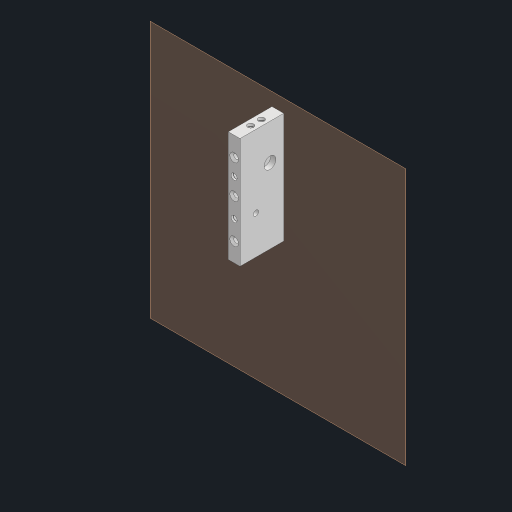
# Autodesk Inventor part: middle_gear_holder
Saved by Autodesk Inventor 2023 (Build 270158000, 158)
## iProperties
Created: 2024-04-23
Part Number: middle_gear_holder
Material: Generic
Document SubType Name: Modeling
Designer: szymo
Density: 1 g/cm^3
Appearance: Default
Author: szymo
Autodesk Inventor part; units mm, degrees
ref_plane "YZ Plane" through (0, 0, 0) normal (1, 0, 0) x (0, 1, 0)
ref_plane "XZ Plane" through (0, 0, 0) normal (0, 1, 0) x (-1, 0, 0)
ref_plane "Work Plane1" through (0, 0, 0) normal (0, 0, 1) x (1, 0, 0)
ref_plane "Work Plane2" through (-89, -40.3889, 33.5) normal (0, 0, 1) x (1, 0, 0)
sketch "Sketch1" plane through (0, 0, 0) normal (0, 0, 1) x (1, 0, 0)
  line L0 (23.5, 88.5) -> (-23.5, 88.5) projected
  line L1 (-23.5, 88.5) -> (-23.5, 36.5) projected
  line L2 (-26.5, 33.5) -> (-89, 33.5) projected
  line L3 (-89, 33.5) -> (-89, -72.5) projected
  line L4 (-89, -72.5) -> (-77, -72.5) projected
  line L5 (-74, -75.5) -> (-74, -93.5) projected
  line L6 (-74, -93.5) -> (74, -93.5) projected
  line L7 (74, -93.5) -> (74, -75.5) projected
  line L8 (77, -72.5) -> (89, -72.5) projected
  line L9 (89, -72.5) -> (89, 33.5) projected
  line L10 (89, 33.5) -> (26.5, 33.5) projected
  line L11 (23.5, 36.5) -> (23.5, 88.5) projected
  line L12 (-4.5, 81.5) -> (-4.5, 36.5) projected
  line L13 (-7.5, 33.5) -> (-13.5, 33.5) projected
  line L14 (-16.5, 36.5) -> (-16.5, 81.5) projected
  line L15 (-13.5, 84.5) -> (-7.5, 84.5) projected
  line L16 (16.5, 81.5) -> (16.5, 36.5) projected
  line L17 (13.5, 33.5) -> (7.5, 33.5) projected
  line L18 (4.5, 36.5) -> (4.5, 81.5) projected
  line L19 (7.5, 84.5) -> (13.5, 84.5) projected
  line L20 (-4.5, 88.5) -> (4.5, 88.5)
  line L21 (4.5, 88.5) -> (4.5, 3.75)
  line L22 (4.5, 3.75) -> (-4.5, 3.75)
  line L23 (-4.5, 3.75) -> (-4.5, 88.5)
  line L24 (-32.2, 4.75) -> (-59.9, 4.75)
  arc A0 (13.5, 33.5) -> (16.5, 36.5) centre (13.5, 36.5) ccw projected
  arc A1 (4.5, 36.5) -> (7.5, 33.5) centre (7.5, 36.5) ccw projected
  arc A2 (7.5, 84.5) -> (4.5, 81.5) centre (7.5, 81.5) ccw projected
  arc A3 (16.5, 81.5) -> (13.5, 84.5) centre (13.5, 81.5) ccw projected
  arc A4 (-4.5, 81.5) -> (-7.5, 84.5) centre (-7.5, 81.5) ccw projected
  arc A5 (-7.5, 33.5) -> (-4.5, 36.5) centre (-7.5, 36.5) ccw projected
  arc A6 (-16.5, 36.5) -> (-13.5, 33.5) centre (-13.5, 36.5) ccw projected
  arc A7 (-13.5, 84.5) -> (-16.5, 81.5) centre (-13.5, 81.5) ccw projected
  arc A8 (-26.5, 33.5) -> (-23.5, 36.5) centre (-26.5, 36.5) ccw projected
  arc A9 (-74, -75.5) -> (-77, -72.5) centre (-77, -75.5) ccw projected
  arc A10 (77, -72.5) -> (74, -75.5) centre (77, -75.5) ccw projected
  arc A11 (23.5, 36.5) -> (26.5, 33.5) centre (26.5, 36.5) ccw projected
  point P0 (0, 0)
  point P1 (-4.5, 81.5)
  point P2 (-4.5, 36.5)
  dimension "d0" = 1
  constraints: 10 end point, 2 collinear, 2 horizontal, 2 parallel, 1 perpendicular, 1 point on line, 2 other
  measures "d0" distance between parallel lines of L24 L22
extrude "Extrusion1" add sketch "Sketch1" along normal up to surface (33.5 mm away) contours L21 L18 L22 L23 L12 L0
sketch "Sketch2" plane through (4.5, 3.75, 0) normal (1, 0, 0) x (0, 0, -1)
  circle A0 centre (-21.2694, 29.2497) radius 2 projected
  point P0 (0, -3.75)
extrude "Extrusion2" cut sketch "Sketch2" against normal blind 10
sketch "Sketch3" plane through (4.5, 3.75, 0) normal (1, 0, 0) x (0, 0, -1)
  circle A0 centre (-10.5, 57.25) radius 4.5 projected
  point P0 (0, -3.75)
extrude "Extrusion3" cut sketch "Sketch3" against normal blind 4
sketch "Sketch4" plane through (-4.5, 3.75, 0) normal (-1, 0, 0) x (0, 0, 1)
  circle A0 centre (10.5, 57.25) radius 4.5 projected
  point P0 (0, -3.75)
extrude "Extrusion4" cut sketch "Sketch4" against normal blind 4
sketch "Sketch5" plane through (-4.5, 3.75, 33.5) normal (0, 0, 1) x (1, 0, 0)
  line L0 (5, 61.75) -> (5, 52.75) projected
  line L1 (4, 52.75) -> (4, 61.75) projected
  line L2 (9, 27.2497) -> (0, 27.2497) projected
  line L3 (9, 31.2497) -> (0, 31.2497) projected
  line L4 (17, 78.15) -> (-8, 78.15)
  line L5 (-8, 35.85) -> (17, 35.85)
  line L6 (9, 84.75) -> (9, 0) projected
  line L7 (0, 52.75) -> (0, 61.75) projected
  line L8 (9, 35.85) -> (0, 35.85)
  line L9 (0, 35.85) -> (0, 52.75)
  line L10 (0, 52.75) -> (9, 52.75)
  line L11 (9, 52.75) -> (9, 35.85)
  line L12 (0, 0) -> (0, 84.75) projected
  line L13 (9, 78.15) -> (0, 78.15)
  line L14 (0, 78.15) -> (0, 61.75)
  line L15 (0, 61.75) -> (9, 61.75)
  line L16 (9, 61.75) -> (9, 78.15)
  line L17 (-18, 7.625) -> (-18, 21.125) projected
  line L18 (-18, 14.375) -> (27, 14.375)
  line L19 (9, 35.85) -> (0, 52.75)
  line L20 (9, 61.75) -> (9, 52.75) projected
  line L21 (0, 35.85) -> (9, 52.75)
  line L22 (9, 61.75) -> (0, 78.15)
  line L23 (0, 61.75) -> (9, 78.15)
  point P0 (4.5, -3.75)
  point P1 (4.5, 14.375)
  point P2 (4.5, 44.3)
  point P3 (4.5, 69.95)
  dimension "d9" = 4.5
  dimension "d10" = 4.5
  constraints: 30 end point, 5 horizontal, 5 point on line, 4 midpoint, 4 parallel, 2 perpendicular, 4 other
  measures "d9" distance from line of L6 point (4.5, 14.375)
  measures "d10" distance from line of point (4.5, 14.375) L12
hole "Hole1" at (0, 18.125, 33.5) at (0, 48.05, 33.5) at (0, 73.7, 33.5) direction (0, 0, -1) diameter 3.6 end through all countersink diameter 6.6 countersink angle 90 clearance for "Countersunk Flat Head Screw ISO 2009/7046" size "M3" standard "ISO"
sketch "Sketch6" plane through (-4.5, 3.75, 0) normal (0, -1, 0) x (1, 0, 0)
  line L0 (9, 33.5) -> (0, 33.5) projected
  line L1 (0, 0) -> (0, 33.5) projected
  line L2 (0, 0) -> (9, 0) projected
  line L3 (9, 0) -> (9, 33.5) projected
  line L4 (0, 16.75) -> (9, 16.75)
  line L5 (9, 16.75) -> (0, 33.5)
  line L6 (9, 33.5) -> (0, 16.75)
  line L7 (0, 16.75) -> (9, 0)
  line L8 (9, 16.75) -> (0, 0)
  point P0 (4.5, 0)
  point P1 (4.5, 8.375)
  point P2 (4.5, 25.125)
  constraints: 10 end point, 4 midpoint, 2 parallel
hole "Hole2" at (0, 3.75, 8.375) at (0, 3.75, 25.125) direction (0, 1, 0) diameter 4 depth 5.35 counterbore diameter 4.6 counterbore depth 0.75
sketch "Sketch7" plane through (-4.5, 88.5, 0) normal (0, 1, 0) x (1, 0, 0)
  line L0 (0, -33.5) -> (9, -33.5) projected
  line L1 (0, -33.5) -> (9, -33.5) projected
  line L2 (9, 0) -> (9, -33.5) projected
  line L3 (9, 0) -> (0, 0) projected
  line L4 (0, 0) -> (0, -33.5) projected
  line L5 (-8, -1.4) -> (-8, -6.6) projected
  line L6 (-8, -32.1) -> (-8, -26.9) projected
  line L7 (17, -32.1) -> (17, -26.9) projected
  line L8 (17, -1.4) -> (17, -6.6) projected
  line L9 (17, -32.1) -> (-8, -32.1)
  line L10 (-8, -32.1) -> (-8, -26.9)
  line L11 (-8, -26.9) -> (17, -26.9)
  line L12 (17, -26.9) -> (17, -32.1)
  line L13 (-8, -6.6) -> (17, -6.6)
  line L14 (17, -6.6) -> (17, -1.4)
  line L15 (17, -1.4) -> (-8, -1.4)
  line L16 (-8, -1.4) -> (-8, -6.6)
  line L17 (17, -6.6) -> (-8, -6.6)
  line L18 (-8, -6.6) -> (-8, -8.6)
  line L19 (-8, -8.6) -> (17, -8.6)
  line L20 (17, -8.6) -> (17, -6.6)
  line L21 (-8, -26.9) -> (17, -26.9)
  line L22 (17, -26.9) -> (17, -24.9)
  line L23 (17, -24.9) -> (-8, -24.9)
  line L24 (-8, -24.9) -> (-8, -26.9)
  line L25 (9, 0) -> (9, -33.5) projected
  line L26 (9, -16.75) -> (0, -16.75)
  line L27 (0, 0) -> (0, -33.5) projected
  line L28 (9, -24.9) -> (0, -16.75)
  line L29 (9, -8.6) -> (0, -16.75)
  line L30 (0, -8.6) -> (9, -16.75)
  line L31 (9, -16.75) -> (0, -24.9)
  point P0 (4.5, 0)
  point P1 (4.5, -20.825)
  point P2 (4.5, -12.675)
  dimension "d25" = 2
  dimension "d26" = 2
  constraints: 42 end point, 10 point on line, 8 parallel, 5 midpoint, 4 horizontal, 4 perpendicular
  measures "d25" distance of L18.end L17.end
  measures "d26" distance of L22.end L21.end
hole "Hole3" at (0, 88.5, 20.825) at (0, 88.5, 12.675) direction (0, -1, 0) diameter 4 depth 6.5 counterbore diameter 4.6 counterbore depth 2
sketch "Sketch8" plane through (-4.5, 3.75, 33.5) normal (0, 0, 1) x (1, 0, 0)
  line L0 (26, 27.2497) -> (-17, 27.2497)
  line L1 (26, 31.2497) -> (-17, 31.2497)
  line L2 (4, 52.75) -> (-1, 52.75)
  line L3 (4, 61.75) -> (-1, 61.75)
  line L4 (10, 61.75) -> (5, 61.75)
  line L5 (9, 52.75) -> (5, 52.75) projected
  line L6 (0, 0) -> (0, 84.75) projected
  line L7 (9, 52.75) -> (0, 52.75)
  line L8 (0, 52.75) -> (0, 61.75)
  line L9 (0, 61.75) -> (9, 61.75)
  line L10 (9, 61.75) -> (9, 52.75)
  line L11 (9, 27.2497) -> (0, 27.2497) projected
  line L12 (0, 31.2497) -> (9, 31.2497)
  line L13 (9, 31.2497) -> (9, 27.2497)
  line L14 (9, 27.2497) -> (0, 27.2497)
  line L15 (0, 27.2497) -> (0, 31.2497)
  line L16 (9, 27.2497) -> (0, 31.2497)
  line L17 (0, 27.2497) -> (9, 31.2497)
  line L18 (9, 52.75) -> (0, 61.75)
  line L19 (0, 52.75) -> (9, 61.75)
  point P0 (4.5, -3.75)
  point P1 (4.5, 29.2497)
  point P2 (4.5, 57.25)
  constraints: 34 end point, 7 horizontal, 6 point on line, 4 parallel, 3 perpendicular, 2 midpoint, 10 other
hole "Hole4" at (0, 32.9997, 33.5) at (0, 61, 33.5) direction (0, 0, -1) diameter 4 depth 6 counterbore diameter 4.6 counterbore depth 1.5
equation "\"d9\" = d10"
body "Solid1"
